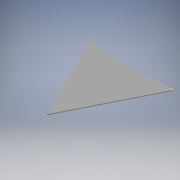
# Autodesk Inventor part: z bELT
Saved by Autodesk Inventor 2018 (Build 220112000, 112)
## iProperties
Created: 2018-05-19
Part Number: z bELT
Material: Generic
Document SubType Name: Modeling
Designer: dan
Density: 1 g/cm^3
Appearance: Default
Author: dan
Autodesk Inventor part; units mm, degrees
ref_plane "YZ Plane" through (0, 0, 0) normal (1, 0, 0) x (0, 1, 0)
ref_plane "XZ Plane" through (0, 0, 0) normal (0, 1, 0) x (-1, 0, 0)
ref_plane "XY Plane" through (0, 0, 0) normal (0, 0, 1) x (1, 0, 0)
sketch "Sketch1" plane through (0, 0, 0) normal (0, 0, 1) x (1, 0, 0)
  arc A0 (-287.0527, -558.563) -> (-272.0536, -558.5587) centre (-279.5531, -558.6452) ccw
  line L0 (-561.7795, -4.4916) -> (-287.0527, -558.563)
  line L1 (-272.0536, -558.5587) -> (6.4474, -0.1094)
  line L2 (-0.0123, 6.4539) -> (-558.6713, 5.3904)
  arc A1 (-558.6713, 5.3904) -> (-561.7795, -4.4916) centre (-558.6609, -0.0427) ccw
  arc A2 (6.4474, -0.1094) -> (-0.0123, 6.4539) centre (1.1622, 1.1493) ccw
  point P0 (0, 0)
  dimension "d0" = 5.433
  constraints: 6 end point, 6 point on circle, 3 centre point, 1 tangent
  measures "d0" radius of A2
extrude "Extrusion1" add sketch "Sketch1" along normal blind 6
sketch "Sketch3" plane through (0, 0, 6) normal (0, 0, 1) x (1, 0, 0)
  line L0 (-561.7795, -4.4916) -> (-287.0527, -558.563) projected
  arc A0 (-287.0527, -558.563) -> (-272.0536, -558.5587) centre (-279.5531, -558.6452) ccw projected
  line L1 (-272.0536, -558.5587) -> (6.4474, -0.1094) projected
  arc A1 (6.4474, -0.1094) -> (-0.0123, 6.4539) centre (1.1622, 1.1493) ccw projected
  line L2 (-0.0123, 6.4539) -> (-558.6713, 5.3904) projected
  arc A2 (-558.6713, 5.3904) -> (-561.7795, -4.4916) centre (-558.6609, -0.0427) ccw projected
  line L3 (-0.0123, 6.4539) -> (-279.291, -20.76)
  line L4 (-0.0123, 6.4539) -> (-558.6713, 5.3904) projected
  line L5 (-279.291, -20.76) -> (-558.6713, 5.3904)
  line L6 (-558.6713, 5.3904) -> (-279.551, 142.5192)
  line L7 (-279.551, 142.5192) -> (-0.0123, 6.4539)
  point P0 (0, 0)
  constraints: 8 end point, 1 point on line
extrude "Extrusion2" cut sketch "Sketch3" against normal blind 6 contours L6 L7 L2 | L2 L3 L5
sketch "Sketch4" plane through (0, 0, 6) normal (0, 0, 1) x (1, 0, 0)
  point P0 (0, 0)
sketch "Sketch5" plane through (0, 0, 6) normal (0, 0, 1) x (1, 0, 0)
  line L0 (-0.0123, 6.4539) -> (-279.291, -20.76) projected
  line L1 (-279.291, -20.76) -> (-558.6713, 5.3904) projected
  arc A0 (-558.6713, 5.3904) -> (-561.7795, -4.4916) centre (-558.6609, -0.0427) ccw projected
  line L2 (-561.7795, -4.4916) -> (-287.0527, -558.563) projected
  arc A1 (-287.0527, -558.563) -> (-272.0536, -558.5587) centre (-279.5531, -558.6452) ccw projected
  line L3 (-272.0536, -558.5587) -> (6.4474, -0.1094) projected
  arc A2 (6.4474, -0.1094) -> (-0.0123, 6.4539) centre (1.1622, 1.1493) ccw projected
  arc A3 (-285.3025, -558.563) -> (-273.8037, -558.563) centre (-279.5531, -558.6452) ccw
  arc A4 (5.0344, -1.1313) -> (0.2947, 5.5587) centre (1.1622, 1.1493) ccw
  arc A5 (-558.1379, 4.3653) -> (-560.7286, -3.9705) centre (-558.6609, -0.0427) ccw
  line L4 (-560.7286, -3.9705) -> (-285.3025, -558.563)
  line L5 (-273.8037, -558.563) -> (5.0344, -1.1313)
  line L6 (1.1622, 5.6432) -> (-279.5531, -21.7107)
  line L7 (-279.5531, -21.7107) -> (-558.1379, 4.3653)
  point P0 (0, 0)
  dimension "d5" = 11.5
  constraints: 8 end point, 7 point on circle, 3 centre point, 3 coincident, 2 parallel, 1 point on line
  measures "d5" diameter of A3
extrude "Extrusion3" cut sketch "Sketch5" against normal blind 6 contours L4 A5 L7 L6 A4 L5 A3
body "Solid1"
